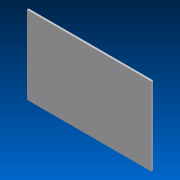
# Autodesk Inventor part: side face
Saved by Autodesk Inventor 2012 (Build 160160000, 160)
## iProperties
Created: 2012-07-02
Part Number: side face
Material: Default
Document SubType Name: Modeling
Designer: Hemant
Density: 1 g/cm^3
Author: Hemant
Autodesk Inventor part; units mm, degrees
ref_plane "YZ Plane" through (0, 0, 0) normal (1, 0, 0) x (0, 1, 0)
ref_plane "XZ Plane" through (0, 0, 0) normal (0, 1, 0) x (-1, 0, 0)
ref_plane "XY Plane" through (0, 0, 0) normal (0, 0, 1) x (1, 0, 0)
sketch "Sketch1" plane through (0, 0, 0) normal (0, 0, 1) x (1, 0, 0)
  line L0 (425.45, 266.7) -> (0, 266.7)
  line L1 (0, 266.7) -> (0, 0)
  line L2 (0, 0) -> (425.45, 0)
  line L3 (425.45, 0) -> (425.45, 266.7)
  dimension "d0" = 425.45
  dimension "d1" = 266.7
  constraints: 8 end point, 2 parallel, 1 horizontal, 1 perpendicular
  measures "d0" distance between parallel lines of L3 L1
  measures "d1" distance between parallel lines of L0 L2
extrude "Extrusion1" add sketch "Sketch1" against normal blind 6.35
body "Solid1"
